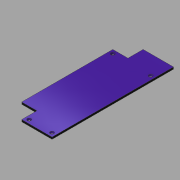
# Autodesk Inventor part: STARduino layout
Saved by Autodesk Inventor 2017 (Build 210142000, 142)
## iProperties
Created: 2017-01-15
Part Number: STARduino layout
Material: Generic
Document SubType Name: Modeling
Designer: qupec
Density: 1 g/cm^3
Appearance: Default
Author: qupec
Autodesk Inventor part; units mm, degrees
ref_plane "YZ Plane" through (0, 0, 0) normal (1, 0, 0) x (0, 1, 0)
ref_plane "XZ Plane" through (0, 0, 0) normal (0, 1, 0) x (-1, 0, 0)
ref_plane "XY Plane" through (0, 0, 0) normal (0, 0, 1) x (1, 0, 0)
sketch "Sketch1" plane through (0, 0, 0) normal (0, 1, 0) x (-1, 0, 0)
  line L0 (19.05, 38.1) -> (6.35, 38.1)
  line L1 (6.35, -38.1) -> (19.05, -38.1)
  line L2 (19.05, -38.1) -> (19.05, 38.1)
  line L3 (6.35, 50.8) -> (-19.05, 50.8)
  line L4 (-19.05, 50.8) -> (-19.05, -50.8)
  line L5 (-19.05, -50.8) -> (6.35, -50.8)
  line L6 (6.35, -50.8) -> (6.35, -38.1)
  line L7 (6.35, 38.1) -> (6.35, 50.8)
  point P0 (0, 0)
  dimension "d0" = 76.2
  dimension "d2" = 101.6
  dimension "d3" = 12.7
  dimension "d4" = 12.7
  dimension "d5" = 25.4
  dimension "d6" = 12.7
  dimension "d7" = 50.8
  dimension "d8" = 38.1
  dimension "d9" = 19.05
  dimension "d10" = 12.7
  constraints: 16 end point, 4 parallel, 2 horizontal, 1 perpendicular
  measures "d0" distance of L1.end L0.start
  measures "d2" distance of L3.end L4.end
  measures "d3" distance between parallel lines of L0 L3
  measures "d4" distance of L0.start L0.end
  measures "d5" distance of L3.start L3.end
  measures "d6" distance of L5.end L1.start
  measures "d7" distance from line of point (0, 0) L3
  measures "d8" horizontal distance of L4.end L1.end
  measures "d9" distance from line of point (0, 0) L2
  measures "d10" distance of L1.start L1.end
extrude "Extrusion1" add sketch "Sketch1" along normal blind 1.651
sketch "Sketch2" plane through (0, 1.651, 0) normal (0, 1, 0) x (1, 0, 0)
  circle A0 centre (-3.175, -47.625) radius 1.5875
  circle A1 centre (15.875, -47.625) radius 1.5875
  circle A2 centre (-15.875, 34.925) radius 1.5875
  circle A3 centre (15.875, 34.925) radius 1.5875
  line L0 (-6.35, 38.1) -> (-19.05, 38.1) projected
  line L1 (-19.05, 38.1) -> (-19.05, -38.1) projected
  line L2 (19.05, -50.8) -> (19.05, 50.8) projected
  line L3 (-6.35, -50.8) -> (19.05, -50.8) projected
  line L4 (-6.35, -38.1) -> (-6.35, -50.8) projected
  point P0 (0, 0)
  dimension "d13" = 3.175
  dimension "d14" = 3.175
  dimension "d15" = 3.175
  dimension "d16" = 3.175
  dimension "d17" = 3.175
  dimension "d18" = 3.175
  dimension "d19" = 3.175
  dimension "d20" = 3.175
  dimension "d21" = 3.175
  dimension "d22" = 3.175
  dimension "d23" = 3.175
  dimension "d24" = 3.175
  constraints: 4 centre point
  measures "d13" diameter of A2
  measures "d14" diameter of A3
  measures "d15" diameter of A0
  measures "d16" diameter of A1
  measures "d17" distance from line of L0 A2.centre
  measures "d18" distance from line of L1 A2.centre
  measures "d19" distance from line of L2 A3.centre
  measures "d20" distance from line of L0 A3.centre
  measures "d21" distance from line of L2 A1.centre
  measures "d22" distance from line of L3 A1.centre
  measures "d23" distance from line of L3 A0.centre
  measures "d24" distance from line of L4 A0.centre
extrude "Extrusion2" cut sketch "Sketch2" against normal through all
equation "\"d6\" = d3"
equation "\"d7\" = 0.5 * d2"
equation "\"d9\" = 0.5 * d8"
equation "\"d10\" = d4"
equation "\"d14\" = d13"
equation "\"d15\" = d13"
equation "\"d16\" = d13"
equation "\"d19\" = d18"
equation "\"d20\" = d17"
equation "\"d21\" = d19"
equation "\"d22\" = d17"
equation "\"d23\" = d17"
equation "\"d24\" = d18"
body "Solid1"
